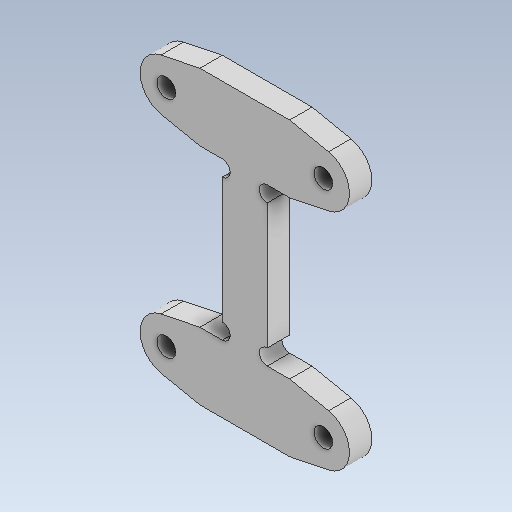
# Autodesk Inventor part: シールド根本留め具
Saved by Autodesk Inventor 2020 (Build 240168000, 168)
## iProperties
Created: 2020-02-05
Part Number: シールド根本留め具
Material: 一般
Document SubType Name: Modeling
Designer: tanjihayato
Density: 1 g/cm^3
Appearance: 既定
Mass: 1.6136 g
Surface Area: 16.6082 cm^2
Volume: 1.6136 cm^3
Author: tanjihayato
Autodesk Inventor part; units mm, degrees
ref_plane "YZ Plane" through (0, 0, 0) normal (1, 0, 0) x (0, 1, 0)
ref_plane "XZ Plane" through (0, 0, 0) normal (0, 1, 0) x (-1, 0, 0)
ref_plane "XY Plane" through (0, 0, 0) normal (0, 0, 1) x (1, 0, 0)
sketch "スケッチ1" plane through (0, 0, 0) normal (0, 0, 1) x (1, 0, 0)
  line L0 (0, 0) -> (6, 0)
  line L1 (6, 0) -> (6, -39)
  line L2 (6, -39) -> (0, -39)
  line L3 (0, -39) -> (0, 0)
  line L4 (6, 0) -> (9, 0)
  circle A0 centre (13.5, -4.5) radius 1.25
  circle A1 centre (-7.5, -4.5) radius 1.25
  circle A2 centre (-7.5, -34.5) radius 1.25
  circle A3 centre (13.5, -34.5) radius 1.25
  circle A4 centre (-7.5, -4.5) radius 3.5
  circle A5 centre (13.5, -4.5) radius 3.5
  circle A6 centre (13.5, -34.5) radius 3.5
  circle A7 centre (-7.5, -34.5) radius 3.5
  line L5 (0, 0) -> (-3, 0)
  line L6 (-3, 0) -> (-8.2059, -1.0719)
  line L7 (-8.2059, -7.9281) -> (-3, -9)
  line L8 (-3, -9) -> (0, -9)
  line L9 (6, -9) -> (9, -9)
  line L10 (9, -9) -> (14.2059, -7.9281)
  line L11 (14.2059, -31.0719) -> (9, -30)
  line L12 (9, -30) -> (6, -30)
  line L13 (0, -30) -> (-3, -30)
  line L14 (-3, -30) -> (-8.2059, -31.0719)
  line L15 (-8.2059, -37.9281) -> (-3, -39)
  line L16 (-3, -39) -> (0, -39)
  line L17 (6, -39) -> (9, -39)
  line L18 (9, -39) -> (14.2059, -37.9281)
  line L19 (-7.5, -34.5) -> (13.5, -34.5) construction
  line L20 (9, 0) -> (14.2059, -1.0719)
  circle A8 centre (0, -10.05) radius 1.05
  circle A9 centre (6, -10.05) radius 1.05
  circle A10 centre (0, -28.95) radius 1.05
  circle A11 centre (6, -28.95) radius 1.05
  point P0 (0, -9)
  point P1 (0, -11.1)
  point P2 (0, -27.9)
  point P3 (6, -27.9)
  point P4 (6, -11.1)
  dimension "d0" = 6
  dimension "d1" = 39
  dimension "d2" = 3
  dimension "d3" = 2.5
  dimension "d4" = 2.5
  dimension "d5" = 2.5
  dimension "d6" = 2.5
  dimension "d7" = 7
  dimension "d8" = 7
  dimension "d9" = 7
  dimension "d10" = 7
  dimension "d11" = 3
  dimension "d12" = 3
  dimension "d13" = 3
  dimension "d14" = 3
  dimension "d15" = 3
  dimension "d16" = 3
  dimension "d19" = 4.5
  dimension "d20" = 4.5
  dimension "d21" = 7.5
  dimension "d22" = 7.5
  dimension "d23" = 3
  dimension "d24" = 7.5
  dimension "d25" = 4.5
  dimension "d26" = 7.5
  dimension "d27" = 4.5
  dimension "d28" = 2.1
  dimension "d29" = 2.1
  dimension "d30" = 2.1
  dimension "d31" = 2.1
  constraints: 42 end point, 12 centre point, 12 point on line, 11 tangent, 8 point on circle, 6 perpendicular, 4 coincident, 4 horizontal, 3 parallel
  measures "d0" distance of L0.start L0.end
  measures "d1" distance of L0.end L1.end
  measures "d2" distance of L0.end L4.end
  measures "d3" diameter of A0
  measures "d4" diameter of A1
  measures "d5" diameter of A2
  measures "d6" diameter of A3
  measures "d7" diameter of A4
  measures "d8" diameter of A5
  measures "d9" diameter of A6
  measures "d10" diameter of A7
  measures "d11" distance of L0.start L5.end
  measures "d12" distance of L9.start L9.end
  measures "d13" distance of L13.start L13.end
  measures "d14" distance of L15.end L2.end
  measures "d15" distance of L11.end L12.end
  measures "d16" distance of L1.end L17.end
  measures "d19" distance between parallel lines of L2 L19
  measures "d20" distance between parallel lines of L19 L13
  measures "d21" distance from line of L3 A2.centre
  measures "d22" distance from line of L1 A3.centre
  measures "d23" distance of L7.end L8.end
  measures "d24" distance from line of A1.centre L3
  measures "d25" distance from line of A4.centre L5
  measures "d26" distance from line of L1 A0.centre
  measures "d27" distance from line of L0 A0.centre
  measures "d28" diameter of A8
  measures "d29" diameter of A9
  measures "d30" diameter of A10
  measures "d31" diameter of A11
extrude "押し出し1" add sketch "スケッチ1" along normal blind 3 contours L0 L1 A9 A11 L2 L3 A10 A8 | L3 L8 L7 A4 L6 L5 | L4 L20 A5 L10 L9 L1 | A4 | A5 | L3 L16 L15 A7 L14 L13 | L12 L11 A6 L18 L17 L1 | A7 | A6
